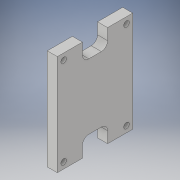
# Autodesk Inventor part: PowerPlugBlockBack
Saved by Autodesk Inventor 2019 (Build 230136000, 136)
## iProperties
Created: 2020-04-21
Part Number: PowerPlugBlockBack
Material: Generic
Document SubType Name: Modeling
Designer: james
Density: 1 g/cm^3
Appearance: Default
Author: james
Autodesk Inventor part; units mm, degrees
ref_plane "YZ Plane" through (0, 0, 0) normal (1, 0, 0) x (0, 1, 0)
ref_plane "XZ Plane" through (0, 0, 0) normal (0, 1, 0) x (-1, 0, 0)
ref_plane "XY Plane" through (0, 0, 0) normal (0, 0, 1) x (1, 0, 0)
sketch "Sketch1" plane through (0, 0, 0) normal (1, 0, 0) x (0, 1, 0)
  line L0 (25.646, 15.8058) -> (-25.154, 15.8058)
  line L1 (-25.154, 15.8058) -> (-25.154, -22.2942)
  line L2 (-25.154, -22.2942) -> (25.646, -22.2942)
  line L3 (25.646, -22.2942) -> (25.646, 15.8058)
  point P0 (0, 0)
  dimension "d0" = 50.8
  dimension "d1" = 38.1
  constraints: 8 end point, 2 parallel, 1 horizontal, 1 perpendicular
  measures "d0" distance of L0.start L0.end
  measures "d1" distance of L2.end L0.start
extrude "Extrusion1" add sketch "Sketch1" along normal blind 5.08
sketch "Sketch2" plane through (5.08, 0, 0) normal (1, 0, 0) x (0, 0, -1)
  line L0 (-15.8058, 25.646) -> (-15.8058, -25.154) projected
  line L1 (22.2942, -25.154) -> (22.2942, 25.646) projected
  line L2 (22.2942, 25.646) -> (-15.8058, 25.646) projected
  line L3 (-15.8058, -25.154) -> (22.2942, -25.154) projected
  point P0 (0, 0)
  point P1 (-12.6308, 22.471)
  point P2 (19.1192, 22.471)
  point P3 (19.1192, -21.979)
  point P4 (-12.6308, -21.979)
  dimension "d4" = 3.175
  dimension "d5" = 0
  dimension "d6" = 3.175
  dimension "d7" = 0
  dimension "d8" = 0
  dimension "d9" = 3.175
  dimension "d10" = 0
  dimension "d11" = 3.175
  measures "d4" distance from line of L0 point (-12.631, 22.471)
  measures "d5" horizontal distance of point (-12.631, -21.979) point (-12.631, 22.471)
  measures "d6" distance from line of L1 point (19.119, 22.471)
  measures "d7" horizontal distance of point (19.119, -21.979) point (19.119, 22.471)
  measures "d8" vertical distance of point (-12.631, 22.471) point (19.119, 22.471)
  measures "d9" distance from line of L2 point (-12.631, 22.471)
  measures "d10" vertical distance of point (19.119, -21.979) point (-12.631, -21.979)
  measures "d11" distance from line of L3 point (-12.631, -21.979)
hole "Hole1" at (5.08, 22.471, 12.6308) at (5.08, 22.471, -19.1192) at (5.08, -21.979, -19.1192) at (5.08, -21.979, 12.6308) direction (-1, 0, 0) diameter 2.794 end through all clearance for "Flat Head Machine Screw (82)" size "#3" standard "Ansi Unified Screw Threads"
sketch "Sketch3" plane through (5.08, 0, 0) normal (1, 0, 0) x (0, 0, -1)
  line L0 (-3.1058, 25.646) -> (9.5942, 25.646)
  line L1 (9.5942, 25.646) -> (9.5942, 19.931)
  line L2 (6.4192, 16.756) -> (0.0692, 16.756)
  line L3 (-3.1058, 19.931) -> (-3.1058, 25.646)
  line L4 (0.0692, -16.264) -> (6.4192, -16.264)
  line L5 (9.5942, -19.439) -> (9.5942, -25.154)
  line L6 (9.5942, -25.154) -> (-3.1058, -25.154)
  line L7 (-3.1058, -25.154) -> (-3.1058, -19.439)
  line L8 (22.2942, 25.646) -> (-15.8058, 25.646) projected
  line L9 (-15.8058, -25.154) -> (22.2942, -25.154) projected
  line L10 (22.2942, -25.154) -> (22.2942, 25.646) projected
  line L11 (-15.8058, 25.646) -> (-15.8058, -25.154) projected
  arc A0 (-3.1058, 19.931) -> (0.0692, 16.756) centre (0.0692, 19.931) ccw
  arc A1 (6.4192, 16.756) -> (9.5942, 19.931) centre (6.4192, 19.931) ccw
  arc A2 (9.5942, -19.439) -> (6.4192, -16.264) centre (6.4192, -19.439) ccw
  arc A3 (0.0692, -16.264) -> (-3.1058, -19.439) centre (0.0692, -19.439) ccw
  point P0 (0, 0)
  point P1 (9.5942, 16.756)
  point P2 (-3.1058, 16.756)
  point P3 (-3.1058, -16.264)
  point P4 (9.5942, -16.264)
  dimension "d19" = 0
  dimension "d20" = 0
  dimension "d21" = 0
  dimension "d22" = 0
  dimension "d23" = 12.7
  dimension "d24" = 12.7
  dimension "d25" = 8.89
  dimension "d26" = 8.89
  dimension "d29" = 3.175
  constraints: 16 end point, 8 point on circle, 8 point on line, 8 tangent, 4 centre point, 4 parallel, 3 equal radius, 2 horizontal, 2 perpendicular
  measures "d19" distance between parallel lines of L8 L0
  measures "d20" distance between parallel lines of L9 L6
  measures "d21" distance between parallel lines of L3 L7
  measures "d22" distance between parallel lines of L5 L1
  measures "d23" distance between parallel lines of L10 L1
  measures "d24" distance between parallel lines of L11 L3
  measures "d25" distance between parallel lines of L6 L4
  measures "d26" distance between parallel lines of L0 L2
  measures "d29" radius of A0
extrude "Extrusion2" cut sketch "Sketch3" against normal blind 20.6375 contours L0 L1 A1 L2 A0 L3 | L7 A3 L4 A2 L5 L6
body "Solid1"
